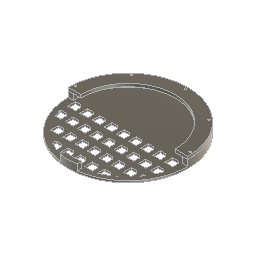
Drip Tray v5 (Autodesk Fusion 360 design; units mm, degrees)
Autodesk Fusion 360 part; units mm, degrees
note: some values were not read from the file. Set by a fixed rule: which sketch regions a step uses.
sketch "Sketch1" plane through (0, 0, 0) normal (0, 0, 1) x (1, 0, 0)
  circle A0 centre (0, 0) radius 56.5
  circle A1 centre (0, 0) radius 61.5
  line L0 (0, 0) -> (0, 131.5) construction
  line L1 (0, 131.5) -> (-54.3597, 28.7624) construction
  line L2 (0, 131.5) -> (54.3597, 28.7624) construction
  line L3 (0, 131.5) -> (89.5717, 41.9283)
  line L4 (0, 131.5) -> (126.6735, 131.5) construction
  line L5 (0, 131.5) -> (-89.2315, 42.2685)
  line L6 (0, 131.5) -> (-126.1924, 131.5) construction
  line L7 (61.5, 109.178) -> (-61.5, 109.178) construction
  line L8 (-61.5, 109.178) -> (-61.5, -109.178)
  line L9 (-61.5, -109.178) -> (61.5, -109.178)
  line L10 (61.5, -109.178) -> (61.5, 109.178)
  line L11 (61.5, 109.178) -> (-61.5, -109.178) construction
  line L12 (-61.5, 109.178) -> (61.5, -109.178) construction
  line L13 (0, 0) -> (0, -61.5) construction
  circle A2 centre (0, -40.75) radius 15.75
  line L14 (4, 0) -> (-4, 0)
  line L15 (-4, 0) -> (-4, -8)
  line L16 (-4, -8) -> (4, -8)
  line L17 (4, -8) -> (4, -2.5)
  line L18 (4, 0) -> (-4, -8) construction
  line L19 (-4, 0) -> (4, -8) construction
  line L20 (4, 0) -> (4, -2.5) construction
  line L21 (4, -2.5) -> (1.5, 0)
  line L22 (-61.5, 0) -> (1.5, 0)
  line L23 (4, 0) -> (61.5, 0)
  line L24 (-46, -2.5) -> (-48.5, 0)
  line L25 (-46, 0) -> (-54, 0)
  line L26 (-54, 0) -> (-54, -8)
  line L27 (-46, -8) -> (-46, -2.5)
  line L28 (-54, -8) -> (-46, -8)
  line L29 (-33.5, -2.5) -> (-36, 0)
  line L30 (-33.5, 0) -> (-41.5, 0)
  line L31 (-41.5, 0) -> (-41.5, -8)
  line L32 (-33.5, -8) -> (-33.5, -2.5)
  line L33 (-41.5, -8) -> (-33.5, -8)
  line L34 (-21, -2.5) -> (-23.5, 0)
  line L35 (-21, 0) -> (-29, 0)
  line L36 (-29, 0) -> (-29, -8)
  line L37 (-21, -8) -> (-21, -2.5)
  line L38 (-29, -8) -> (-21, -8)
  line L39 (-8.5, -2.5) -> (-11, 0)
  line L40 (-8.5, 0) -> (-16.5, 0)
  line L41 (-16.5, 0) -> (-16.5, -8)
  line L42 (-8.5, -8) -> (-8.5, -2.5)
  line L43 (-16.5, -8) -> (-8.5, -8)
  line L44 (16.5, -2.5) -> (14, 0)
  line L45 (16.5, 0) -> (8.5, 0)
  line L46 (8.5, 0) -> (8.5, -8)
  line L47 (16.5, -8) -> (16.5, -2.5)
  line L48 (8.5, -8) -> (16.5, -8)
  line L49 (29, -2.5) -> (26.5, 0)
  line L50 (29, 0) -> (21, 0)
  line L51 (21, 0) -> (21, -8)
  line L52 (29, -8) -> (29, -2.5)
  line L53 (21, -8) -> (29, -8)
  line L54 (41.5, -2.5) -> (39, 0)
  line L55 (41.5, 0) -> (33.5, 0)
  line L56 (33.5, 0) -> (33.5, -8)
  line L57 (41.5, -8) -> (41.5, -2.5)
  line L58 (33.5, -8) -> (41.5, -8)
  line L59 (54, -2.5) -> (51.5, 0)
  line L60 (54, 0) -> (46, 0)
  line L61 (46, 0) -> (46, -8)
  line L62 (54, -8) -> (54, -2.5)
  line L63 (46, -8) -> (54, -8)
  line L64 (-46, -17.5) -> (-48.5, -15)
  line L65 (-46, -15) -> (-54, -15)
  line L66 (-54, -15) -> (-54, -23)
  line L67 (-46, -23) -> (-46, -17.5)
  line L68 (-54, -23) -> (-46, -23)
  line L69 (-33.5, -17.5) -> (-36, -15)
  line L70 (-33.5, -15) -> (-41.5, -15)
  line L71 (-41.5, -15) -> (-41.5, -23)
  line L72 (-33.5, -23) -> (-33.5, -17.5)
  line L73 (-41.5, -23) -> (-33.5, -23)
  line L74 (-21, -17.5) -> (-23.5, -15)
  line L75 (-21, -15) -> (-29, -15)
  line L76 (-29, -15) -> (-29, -23)
  line L77 (-21, -23) -> (-21, -17.5)
  line L78 (-29, -23) -> (-21, -23)
  line L79 (-8.5, -17.5) -> (-11, -15)
  line L80 (-8.5, -15) -> (-16.5, -15)
  line L81 (-16.5, -15) -> (-16.5, -23)
  line L82 (-8.5, -23) -> (-8.5, -17.5)
  line L83 (-16.5, -23) -> (-8.5, -23)
  line L84 (4, -17.5) -> (1.5, -15)
  line L85 (4, -15) -> (-4, -15)
  line L86 (-4, -15) -> (-4, -23)
  line L87 (4, -23) -> (4, -17.5)
  line L88 (-4, -23) -> (4, -23)
  line L89 (16.5, -17.5) -> (14, -15)
  line L90 (16.5, -15) -> (8.5, -15)
  line L91 (8.5, -15) -> (8.5, -23)
  line L92 (16.5, -23) -> (16.5, -17.5)
  line L93 (8.5, -23) -> (16.5, -23)
  line L94 (29, -17.5) -> (26.5, -15)
  line L95 (29, -15) -> (21, -15)
  line L96 (21, -15) -> (21, -23)
  line L97 (29, -23) -> (29, -17.5)
  line L98 (21, -23) -> (29, -23)
  line L99 (41.5, -17.5) -> (39, -15)
  line L100 (41.5, -15) -> (33.5, -15)
  line L101 (33.5, -15) -> (33.5, -23)
  line L102 (41.5, -23) -> (41.5, -17.5)
  line L103 (33.5, -23) -> (41.5, -23)
  line L104 (54, -17.5) -> (51.5, -15)
  line L105 (54, -15) -> (46, -15)
  line L106 (46, -15) -> (46, -23)
  line L107 (54, -23) -> (54, -17.5)
  line L108 (46, -23) -> (54, -23)
  line L109 (-46, -32.5) -> (-48.5, -30)
  line L110 (-46, -30) -> (-54, -30)
  line L111 (-54, -30) -> (-54, -38)
  line L112 (-46, -38) -> (-46, -32.5)
  line L113 (-54, -38) -> (-46, -38)
  line L114 (-33.5, -32.5) -> (-36, -30)
  line L115 (-33.5, -30) -> (-41.5, -30)
  line L116 (-41.5, -30) -> (-41.5, -38)
  line L117 (-33.5, -38) -> (-33.5, -32.5)
  line L118 (-41.5, -38) -> (-33.5, -38)
  line L119 (-21, -32.5) -> (-23.5, -30)
  line L120 (-21, -30) -> (-29, -30)
  line L121 (-29, -30) -> (-29, -38)
  line L122 (-21, -38) -> (-21, -32.5)
  line L123 (-29, -38) -> (-21, -38)
  line L124 (-8.5, -32.5) -> (-11, -30)
  line L125 (-8.5, -30) -> (-16.5, -30)
  line L126 (-16.5, -30) -> (-16.5, -38)
  line L127 (-8.5, -38) -> (-8.5, -32.5)
  line L128 (-16.5, -38) -> (-8.5, -38)
  line L129 (4, -32.5) -> (1.5, -30)
  line L130 (4, -30) -> (-4, -30)
  line L131 (-4, -30) -> (-4, -38)
  line L132 (4, -38) -> (4, -32.5)
  line L133 (-4, -38) -> (4, -38)
  line L134 (16.5, -32.5) -> (14, -30)
  line L135 (16.5, -30) -> (8.5, -30)
  line L136 (8.5, -30) -> (8.5, -38)
  line L137 (16.5, -38) -> (16.5, -32.5)
  line L138 (8.5, -38) -> (16.5, -38)
  line L139 (29, -32.5) -> (26.5, -30)
  line L140 (29, -30) -> (21, -30)
  line L141 (21, -30) -> (21, -38)
  line L142 (29, -38) -> (29, -32.5)
  line L143 (21, -38) -> (29, -38)
  line L144 (41.5, -32.5) -> (39, -30)
  line L145 (41.5, -30) -> (33.5, -30)
  line L146 (33.5, -30) -> (33.5, -38)
  line L147 (41.5, -38) -> (41.5, -32.5)
  line L148 (33.5, -38) -> (41.5, -38)
  line L149 (54, -32.5) -> (51.5, -30)
  line L150 (54, -30) -> (46, -30)
  line L151 (46, -30) -> (46, -38)
  line L152 (54, -38) -> (54, -32.5)
  line L153 (46, -38) -> (54, -38)
  line L154 (-46, -47.5) -> (-48.5, -45)
  line L155 (-46, -45) -> (-54, -45)
  line L156 (-54, -45) -> (-54, -53)
  line L157 (-46, -53) -> (-46, -47.5)
  line L158 (-54, -53) -> (-46, -53)
  line L159 (-33.5, -47.5) -> (-36, -45)
  line L160 (-33.5, -45) -> (-41.5, -45)
  line L161 (-41.5, -45) -> (-41.5, -53)
  line L162 (-33.5, -53) -> (-33.5, -47.5)
  line L163 (-41.5, -53) -> (-33.5, -53)
  line L164 (-21, -47.5) -> (-23.5, -45)
  line L165 (-21, -45) -> (-29, -45)
  line L166 (-29, -45) -> (-29, -53)
  line L167 (-21, -53) -> (-21, -47.5)
  line L168 (-29, -53) -> (-21, -53)
  line L169 (-8.5, -47.5) -> (-11, -45)
  line L170 (-8.5, -45) -> (-16.5, -45)
  line L171 (-16.5, -45) -> (-16.5, -53)
  line L172 (-8.5, -53) -> (-8.5, -47.5)
  line L173 (-16.5, -53) -> (-8.5, -53)
  line L174 (4, -47.5) -> (1.5, -45)
  line L175 (4, -45) -> (-4, -45)
  line L176 (-4, -45) -> (-4, -53)
  line L177 (4, -53) -> (4, -47.5)
  line L178 (-4, -53) -> (4, -53)
  line L179 (16.5, -47.5) -> (14, -45)
  line L180 (16.5, -45) -> (8.5, -45)
  line L181 (8.5, -45) -> (8.5, -53)
  line L182 (16.5, -53) -> (16.5, -47.5)
  line L183 (8.5, -53) -> (16.5, -53)
  line L184 (29, -47.5) -> (26.5, -45)
  line L185 (29, -45) -> (21, -45)
  line L186 (21, -45) -> (21, -53)
  line L187 (29, -53) -> (29, -47.5)
  line L188 (21, -53) -> (29, -53)
  line L189 (41.5, -47.5) -> (39, -45)
  line L190 (41.5, -45) -> (33.5, -45)
  line L191 (33.5, -45) -> (33.5, -53)
  line L192 (41.5, -53) -> (41.5, -47.5)
  line L193 (33.5, -53) -> (41.5, -53)
  line L194 (54, -47.5) -> (51.5, -45)
  line L195 (54, -45) -> (46, -45)
  line L196 (46, -45) -> (46, -53)
  line L197 (54, -53) -> (54, -47.5)
  line L198 (46, -53) -> (54, -53)
  line L199 (-8.5, -60.9098) -> (-8.5, -55.857)
  line L200 (8.5, -60.9098) -> (8.5, -55.857)
  point P0 (0, -4)
  dimension "d1" = 113
  dimension "d2" = 5
  dimension "d7" = 131.5
  dimension "d8" = 45
  dimension "d9" = 45
  dimension "d10" = 123
  dimension "d16" = 8
  dimension "d17" = 8
  dimension "d18" = 2.5
  dimension "d21" = 50
  dimension "d22" = -45
  constraint coincident A0.centre A1.centre
  constraint vertical L0
  constraint coincident A1 L1.end
  constraint tangent A1 L1
  constraint coincident A1 L2.end
  constraint tangent A1 L2
  constraint horizontal L4
  constraint horizontal L6
  constraint horizontal L7
  constraint perpendicular L7 L8
  constraint parallel L7 L9
  constraint parallel L8 L10
  constraint coincident L11 A0.centre
  constraint coincident L12 A0.centre
  constraint midpoint L8 L22.start
  constraint midpoint L10 L23.end
  constraint coincident A1 L13.end
  constraint parallel L0 L13
  constraint horizontal L14
  constraint perpendicular L14 L15
  constraint parallel L14 L16
  constraint parallel L15 L17
  constraint coincident L14.start L22
  constraint coincident L18 P0
  constraint coincident L19 P0
  constraint coincident L13 P0
  constraint collinear L22 L23
  constraint coincident A1 L199.start
  constraint coincident A0 L199.end
  constraint parallel L172 L199
  constraint coincident A1 L200.start
  constraint coincident A0 L200.end
  constraint vertical L200
  measures "d1" diameter of A0
  measures "d7" distance of A0.centre L0.end
  measures "d8" angle of L3 L4
  measures "d9" angle of L5 L6
  measures "d10" distance of L8.end L9.end
  measures "d16" distance of L15.end L16.end
  measures "d17" distance of L14.end L15.end
  measures "d18" vertical distance of L17.end L21.end
extrude "Extrude1" add sketch "Sketch1" against normal blind 2 contours A0 L14 L22 L23 L25 L30 L35 L40 L45 L50 L55 L60 | A0 A1 L23 L104 L107 L108 L150 | A2 L124 L125 L127 L128 L135 L136 L138 L169 L170 L172 L173 L180 L181 L183 | A0 L14 L15 L16 L17 L21 L22 L23 L24 L25 L26 L27 L28 L29 L30 L31 L32 L33 L34 L35 L36 L37 L38 L39 L40 L41 L42 L43 L44 L45 L46 L47 L48 L49 L50 L51 L52 L53 L54 L55 L56 L57 L58 L59 L60 L61 L62 L63 L64 L65 L66 L67 L68 L104 L105 L106 L108 L109 L112 L150 L151 L164 L165 L166 L167 L184 L185 L186 L187 L190 L191 | A0 A1 L22 L23 | A0 A1 L22 L66 L68 L110 | A0 L104 L107 L108 | A0 L66 L68 | A1 L149 L150 | A0 A1 L109 L110 L112 L113 | A0 A1 L149 L150 L151 L153 | A0 L109 L110 | A0 A1 L112 L113 L160 L161 | A0 A1 L151 L153 L189 L190 | A0 L109 L112 | A1 L159 L160 L161 L162 | A0 A1 L189 L190 L191 | A0 A1 L159 L160 L162 L166 L167 L168 L199 | A0 A1 L186 L187 L188 L191 L200 | A0 A1 L199 L200 | A0 L186 L187 L188 | A0 L166 L167 L168 makes body 1
extrude "Extrude2" add sketch "Sketch1" along normal blind 6 contours A0 A1 L22 L23 | A0 A1 L199 L200 bodies 1
sketch "Sketch2" plane through (0, 0, 6) normal (0, 0, 1) x (-1, 0, 0)
  arc A0 (-61.5, 0) -> (61.5, 0) centre (0, 0) ccw
  line L0 (-56.5, 0) -> (-61.5, 0)
  arc A1 (-56.5, 0) -> (56.5, 0) centre (0, 0) ccw
  line L1 (-69.038, -8) -> (-47.8357, -8)
  arc A2 (47.8357, -8) -> (-47.8357, -8) centre (0, 0) ccw
  line L2 (47.8357, -8) -> (69.038, -8)
  arc A3 (69.038, -8) -> (-69.038, -8) centre (0, 0) ccw
  line L3 (61.5, 0) -> (-1.5, 0)
  line L4 (-61.5, 0) -> (-80, 0)
  line L5 (-80, 0) -> (-56.5, 0)
  line L6 (-56.5, 0) -> (69.5, 0)
  arc A4 (-69.5, 0) -> (69.038, 8) centre (0, 0) ccw
  line L7 (69.038, 8) -> (47.8357, 8)
  arc A5 (-48.5, 0) -> (47.8357, 8) centre (0, 0) ccw
  line L8 (61.5, 0) -> (56.5, 0)
  constraint parallel L0 L1
  constraint concentric A1 A2
  constraint concentric A0 A3
  constraint coincident A0.start L0.end
  constraint parallel L0 L4
  constraint coincident L0.start A1.start
  constraint parallel L0 L5
  constraint coincident A3 L6.end
  constraint parallel L4 L6
  constraint concentric A0 A4
  constraint concentric A1 A5
extrude "Extrude3" add sketch "Sketch2" along normal blind 3 separate body contours A0 L0 A1 L1 L5 | A0 A1 L1 L2 | A1 L1 A2 L6 A5 | A0 A1 L2 L3 L6 L8 | A1 L1 L2 A5 | A1 A2 L2 L3 L6 A5 makes body 2
sketch "Sketch3" plane through (0, 0, 6) normal (0, 0, 1) x (-1, 0, 0)
  line L0 (-56.5, 0) -> (-61.5, 0)
  arc A0 (-61.5, 0) -> (61.5, 0) centre (0, 0) ccw
  line L1 (61.5, 0) -> (56.5, 0)
  arc A1 (-56.5, 0) -> (56.5, 0) centre (0, 0) ccw
  line L2 (0, -61.5) -> (0, -56.5) construction
  circle A2 centre (0, -59) radius 1
  circle A3 centre (-58.7755, -5.1422) radius 1
  circle A4 centre (-39.8598, -43.4994) radius 1
  circle A5 centre (39.8598, -43.4994) radius 1
  circle A6 centre (58.7755, -5.1422) radius 1
  dimension "d24" = 2
  dimension "d26" = 170
  constraint midpoint A0 L2.start
  constraint midpoint A1 L2.end
  constraint midpoint L2 A2.centre
  measures "d24" diameter of A2
extrude "Extrude4" cut sketch "Sketch3" along normal up to surface (3 mm away) and the other way up to surface (7 mm away) contours A2 | A3 | A4 | A5 | A6 bodies 1 2
equation "d7 = 61.500 mm + 70 mm"
named bodies: "drip-tray-base", "drip-tray-top"
